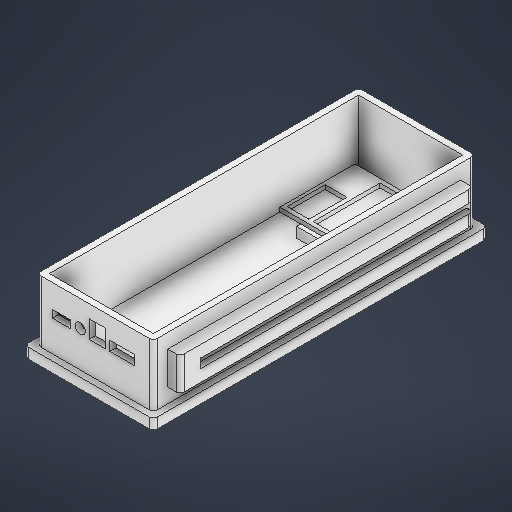
# Autodesk Inventor part: module_command
Saved by Autodesk Inventor 2025.2 (Build 292293000, 293)
## iProperties
Created: 2025-09-05
Part Number: module_command
Material: PC/ABS Plastic
Document SubType Name: Modeling
Designer: sam
Density: 1.1 g/cm^3
Appearance: Smooth - White
Author: sam
Autodesk Inventor part; units mm, degrees
ref_plane "YZ Plane" through (0, 0, 0) normal (1, 0, 0) x (0, 1, 0)
ref_plane "XZ Plane" through (0, 0, 0) normal (0, 1, 0) x (-1, 0, 0)
ref_plane "XY Plane" through (0, 0, 0) normal (0, 0, 1) x (1, 0, 0)
sketch "Sketch1" plane through (0, 0, 0) normal (0, 1, 0) x (-1, 0, 0)
  line L0 (-31.2, -81) -> (31.2, -81)
  line L1 (31.2, -81) -> (31.2, 81)
  line L2 (31.2, 81) -> (-31.2, 81)
  line L3 (-31.2, 81) -> (-31.2, -81)
  line L4 (-31.2, -81) -> (31.2, 81) construction
  line L5 (31.2, -81) -> (-31.2, 81) construction
  point P0 (0, 0)
  dimension "d0" = 62.4
  dimension "d1" = 162
  constraints: 12 end point, 2 midpoint, 2 parallel, 1 horizontal, 1 perpendicular
  measures "d0" distance of L2.end L1.end
  measures "d1" distance of L1.end L0.end
extrude "Extrusion1" add sketch "Sketch1" along normal blind 5
sketch "Sketch2" plane through (0, 5, 0) normal (0, 1, 0) x (1, 0, 0)
  line L0 (-31.2, 81) -> (-31.2, -81) projected
  line L1 (-31.2, -81) -> (31.2, -81) projected
  line L2 (31.2, -81) -> (31.2, 81) projected
  line L3 (31.2, 81) -> (-31.2, 81) projected
  line L4 (28.2, 78) -> (-28.2, 78)
  line L5 (-28.2, 78) -> (-28.2, -78)
  line L6 (-28.2, -78) -> (28.2, -78)
  line L7 (28.2, -78) -> (28.2, 78)
  line L8 (28.2, 78) -> (-28.2, -78) construction
  line L9 (-28.2, 78) -> (28.2, -78) construction
  line L10 (25.2, 75) -> (-25.2, 75)
  line L11 (-25.2, 75) -> (-25.2, -75)
  line L12 (-25.2, -75) -> (25.2, -75)
  line L13 (25.2, -75) -> (25.2, 75)
  line L14 (25.2, 75) -> (-25.2, -75) construction
  line L15 (-25.2, 75) -> (25.2, -75) construction
  point P0 (0, 0)
  dimension "d4" = 3
  dimension "d5" = 3
  dimension "d6" = 3
  dimension "d7" = 3
  constraints: 24 end point, 4 midpoint, 4 parallel, 2 horizontal, 2 perpendicular
  measures "d4" distance between parallel lines of L0 L5
  measures "d5" distance between parallel lines of L1 L6
  measures "d6" distance between parallel lines of L5 L11
  measures "d7" distance between parallel lines of L6 L12
extrude "Extrusion2" add sketch "Sketch2" along normal blind 30 contours L7 L6 L5 L4
fillet "Fillet1" radius 2 4 edges at (-28.2, 20, 78) (28.2, 20, 78) (28.2, 20, -78) (-28.2, 20, -78)
fillet "Fillet2" radius 2 4 edges at (-31.2, 2.5, 81) (31.2, 2.5, 81) (31.2, 2.5, -81) (-31.2, 2.5, -81)
sketch "Sketch3" plane through (28.2, 5, 76) normal (1, 0, 0) x (0, 0, -1)
  line L0 (152, 30) -> (152, 0) projected
  line L1 (0, 30) -> (152, 30) projected
  line L2 (0, 0) -> (0, 30) projected
  line L3 (152, 0) -> (0, 0) projected
  line L4 (5, 23) -> (147, 23)
  line L5 (147, 23) -> (147, 7)
  line L6 (147, 7) -> (5, 7)
  line L7 (5, 7) -> (5, 23)
  line L8 (-2, 30) -> (-2, 0) projected
  line L9 (154, 0) -> (154, 30) projected
  line L10 (157, -5) -> (157, 0) projected
  line L11 (-5, 0) -> (-5, -5) projected
  point P0 (76, -5)
  point P1 (147, 15)
  point P2 (-2, 15)
  dimension "d33" = 16
  dimension "d34" = 8
  dimension "d35" = 10
  dimension "d36" = 10
  constraints: 8 end point, 2 midpoint, 2 parallel, 1 horizontal, 1 perpendicular
  measures "d33" distance between parallel lines of L4 L6
  measures "d34" distance from line of L4 point (-2, 15)
  measures "d35" distance between parallel lines of L10 L5
  measures "d36" distance between parallel lines of L11 L7
extrude "Extrusion3" add sketch "Sketch3" along normal blind 6 contours L4 L5 L6 L7
sketch "Sketch4" plane through (28.2, 12, -71) normal (0, 0, -1) x (-1, 0, 0)
  line L0 (0, 16) -> (0, 0) projected
  line L1 (0, 16) -> (-6, 16) projected
  line L2 (-6, 0) -> (-6, 16) projected
  line L3 (0, 0) -> (-6, 0) projected
  line L4 (-6, 0) -> (-6, 16) projected
  line L5 (0, -7) -> (0, 23) projected
  line L6 (-6, 16) -> (0.4, 16)
  line L7 (0.4, 16) -> (0.4, 13.2)
  line L8 (0.4, 13.2) -> (-6, 13.2)
  line L9 (-6, 13.2) -> (-6, 16)
  line L10 (-6, 0) -> (0.4, 0)
  line L11 (0.4, 0) -> (0.4, 2.8)
  line L12 (0.4, 2.8) -> (-6, 2.8)
  line L13 (-6, 2.8) -> (-6, 0)
  line L14 (-6, 2.8) -> (-3, 2.8)
  line L15 (-3, 2.8) -> (-3, 5.8)
  line L16 (-3, 5.8) -> (-6, 5.8)
  line L17 (-6, 5.8) -> (-6, 2.8)
  line L18 (-6, 13.2) -> (-3, 13.2)
  line L19 (-3, 13.2) -> (-3, 10.2)
  line L20 (-3, 10.2) -> (-6, 10.2)
  line L21 (-6, 10.2) -> (-6, 13.2)
  point P0 (28.2, -12)
  point P1 (-6, 10.2)
  point P2 (-6, 5.8)
  point P3 (-3, 2.8)
  point P4 (0, 2.8)
  point P5 (0, 13.2)
  point P6 (-3, 13.2)
  point P7 (-6, 13.2)
  point P8 (0, 16)
  dimension "d102" = 6.4
  dimension "d103" = 2.8
  dimension "d104" = 6.4
  dimension "d105" = 2.8
  dimension "d106" = 3
  dimension "d107" = 3
  dimension "d108" = 3
  dimension "d109" = 3
  constraints: 32 end point, 8 parallel, 4 horizontal, 4 perpendicular
  measures "d102" distance of L7.end L8.end
  measures "d103" distance of L6.end L7.end
  measures "d104" distance of L12.end L11.end
  measures "d105" distance of L11.end L10.end
  measures "d106" distance of L16.end L15.end
  measures "d107" distance of L15.end L14.end
  measures "d108" distance of L19.end L20.end
  measures "d109" distance of L18.end L19.end
extrude "Extrusion4" cut sketch "Sketch4" against normal blind 132 contours L0 L12 L15 L16 L2 L20 L19 L8
fillet "Fillet3" radius 2 3 edges at (34.2, 20, 71) (34.2, 14.9, -71) (34.2, 25.1, -71)
sketch "Sketch5" plane through (-28.2, 5, -76) normal (-1, 0, 0) x (0, 0, 1)
  line L0 (0, 30) -> (152, 30) projected
  line L1 (-2, 30) -> (-2, 0) projected
  line L2 (154, 0) -> (154, 30) projected
  line L3 (5, 20) -> (137, 20)
  line L4 (137, 20) -> (137, 10)
  line L5 (137, 10) -> (5, 10)
  line L6 (5, 10) -> (5, 20)
  line L7 (-5, 0) -> (-5, -5) projected
  line L8 (157, -5) -> (157, 0) projected
  point P0 (76, -5)
  point P1 (154, 15)
  dimension "d28" = 10
  dimension "d39" = 10
  dimension "d40" = 20
  dimension "d41" = 5
  constraints: 8 end point, 2 parallel, 1 horizontal, 1 midpoint, 1 perpendicular
  measures "d28" distance of L3.end L4.end
  measures "d39" distance between parallel lines of L7 L6
  measures "d40" distance between parallel lines of L8 L4
  measures "d41" distance from line of point (154, 15) L3
extrude "Extrusion5" add sketch "Sketch5" along normal blind 6
sketch "Sketch6" plane through (-28.2, 15, 61) normal (0, 0, 1) x (1, 0, 0)
  line L0 (0, 10) -> (0, 0) projected
  line L1 (0, 10) -> (-6, 10) projected
  line L2 (-6, 0) -> (-6, 10) projected
  line L3 (0, 0) -> (-6, 0) projected
  line L4 (0, 10) -> (-3.4, 10)
  line L5 (-3.4, 10) -> (-3.4, 7)
  line L6 (-3.4, 7) -> (0, 7)
  line L7 (0, 7) -> (0, 10)
  line L8 (0, 0) -> (-3.4, 0)
  line L9 (-3.4, 0) -> (-3.4, 3)
  line L10 (-3.4, 3) -> (0, 3)
  line L11 (0, 3) -> (0, 0)
  point P0 (28.2, -15)
  point P1 (0, 3)
  point P2 (-3.4, 0)
  point P3 (0, 7)
  point P4 (-3.4, 10)
  dimension "d44" = 3.4
  dimension "d45" = 3
  dimension "d46" = 3.4
  dimension "d47" = 3
  constraints: 16 end point, 4 parallel, 2 horizontal, 2 perpendicular
  measures "d44" distance of L6.end L5.end
  measures "d45" distance of L5.end L4.end
  measures "d46" distance of L9.end L10.end
  measures "d47" distance of L8.end L9.end
extrude "Extrusion6" cut sketch "Sketch6" against normal up to surface (132 mm away) contours L0 L6 L5 L1 | L0 L3 L9 L10
fillet "Fillet4" radius 1 18 edges at (-34.2, 25, -5) (-31.6, 25, -5) (-34.2, 15, -5) (-31.6, 15, -5) (-34.2, 20, 61) (-31.6, 23.5, 61) (-32.9, 25, 61) (-32.9, 15, 61) (-31.6, 16.5, 61) (-31.6, 16.5, -71) (-34.2, 20, -71) (-31.6, 23.5, -71) (-32.9, 25, -71) (-32.9, 15, -71) (-29.9, 22, -71) (-29.9, 18, -71) (-29.9, 18, 61) (-29.9, 22, 61)
sketch "Sketch9" plane through (0, 5, 0) normal (0, 1, 0) x (1, 0, 0)
  line L0 (25.2, 75) -> (-25.2, 75) projected
  line L1 (-25.2, 75) -> (-25.2, -75) projected
  line L2 (-25.2, -75) -> (25.2, -75) projected
  line L3 (25.2, -75) -> (25.2, 75) projected
  line L4 (-25.2, -72.6) -> (25.2, -72.6)
  line L5 (25.2, -72.6) -> (25.2, -70.6)
  line L6 (25.2, -70.6) -> (-25.2, -70.6)
  line L7 (-25.2, -70.6) -> (-25.2, -72.6)
  line L8 (-25.2, 75) -> (-25.2, -75) projected
  line L9 (-25.2, 29.8) -> (25.2, 29.8)
  line L10 (25.2, 29.8) -> (25.2, 31.8)
  line L11 (25.2, 31.8) -> (-25.2, 31.8)
  line L12 (-25.2, 31.8) -> (-25.2, 29.8)
  line L13 (-25.2, 31.8) -> (-10.2, 31.8)
  line L14 (-10.2, 31.8) -> (-10.2, 29.8)
  line L15 (-10.2, 29.8) -> (-25.2, 29.8)
  line L16 (-25.2, 29.8) -> (-25.2, 31.8)
  point P0 (0, 0)
  point P1 (25.2, 17.2)
  point P2 (-25.2, 31.8)
  point P3 (25.2, 29.8)
  point P4 (-25.2, -70.6)
  point P5 (-10.2, 31.8)
  dimension "d79" = 2
  dimension "d80" = 2.4
  dimension "d81" = 2
  dimension "d82" = 100.4
  dimension "d87" = 15
  constraints: 24 end point, 6 parallel, 6 point on line, 3 horizontal, 3 perpendicular
  measures "d79" distance of L5.end L4.end
  measures "d80" distance between parallel lines of L2 L4
  measures "d81" distance of L10.end L9.end
  measures "d82" distance between parallel lines of L6 L9
  measures "d87" distance of L14.end L15.end
extrude "Extrusion9" add sketch "Sketch9" along normal blind 5 contours L3 L9 L14 L11 | L3 L4 L1 L6
sketch "Sketch10" plane through (0, 5, 0) normal (0, 1, 0) x (1, 0, 0)
  line L0 (-25.2, -70.6) -> (25.2, -70.6) projected
  line L1 (25.2, -70.6) -> (25.2, 29.8) projected
  line L2 (25.2, 29.8) -> (-10.2, 29.8) projected
  line L3 (-10.2, 29.8) -> (-10.2, 31.8) projected
  line L4 (-10.2, 31.8) -> (25.2, 31.8) projected
  line L5 (25.2, 31.8) -> (25.2, 75) projected
  line L6 (25.2, 75) -> (-25.2, 75) projected
  line L7 (-25.2, 75) -> (-25.2, -70.6) projected
  line L8 (-25.2, 36.8) -> (25.2, 36.8)
  line L9 (-25.2, 71.8) -> (-25.2, 36.8)
  line L10 (-25.2, 36.8) -> (25.2, 36.8)
  line L11 (25.2, 36.8) -> (25.2, 38.8)
  line L12 (25.2, 38.8) -> (-25.2, 38.8)
  line L13 (-25.2, 38.8) -> (-25.2, 36.8)
  line L14 (25.2, 31.8) -> (25.2, 75) projected
  line L15 (-25.2, 38.8) -> (25.2, 38.8)
  line L16 (25.2, 38.8) -> (25.2, 71.2)
  line L17 (25.2, 71.2) -> (-25.2, 71.2)
  line L18 (-25.2, 71.2) -> (25.2, 71.2)
  line L19 (25.2, 71.2) -> (25.2, 73.2)
  line L20 (25.2, 73.2) -> (-25.2, 73.2)
  line L21 (-25.2, 73.2) -> (-25.2, 71.2)
  line L22 (25.2, 38.8) -> (23.7, 38.8)
  line L23 (23.7, 38.8) -> (23.7, 71.2)
  line L24 (23.7, 71.2) -> (25.2, 71.2)
  line L25 (25.2, 71.2) -> (25.2, 38.8)
  line L26 (23.7, 38.8) -> (7.3, 38.8)
  line L27 (7.3, 38.8) -> (7.3, 71.2)
  line L28 (7.3, 71.2) -> (23.7, 71.2)
  line L29 (23.7, 71.2) -> (23.7, 38.8)
  line L30 (7.3, 38.8) -> (5.3, 38.8)
  line L31 (5.3, 38.8) -> (5.3, 71.2)
  line L32 (5.3, 71.2) -> (7.3, 71.2)
  line L33 (7.3, 71.2) -> (7.3, 38.8)
  line L34 (5.3, 38.8) -> (-11.1, 38.8)
  line L35 (-11.1, 38.8) -> (-11.1, 71.2)
  line L36 (-11.1, 71.2) -> (5.3, 71.2)
  line L37 (5.3, 71.2) -> (5.3, 38.8)
  line L38 (-11.1, 38.8) -> (-13.1, 38.8)
  line L39 (-13.1, 38.8) -> (-13.1, 71.2)
  line L40 (-13.1, 71.2) -> (-11.1, 71.2)
  line L41 (-11.1, 71.2) -> (-11.1, 38.8)
  line L42 (-25.2, 71.2) -> (-23.7, 71.2)
  line L43 (-23.7, 71.2) -> (-23.7, 38.8)
  line L44 (-23.7, 38.8) -> (-25.2, 38.8)
  line L45 (-25.2, 38.8) -> (-25.2, 71.2)
  line L46 (-23.7, 38.8) -> (-13.1, 38.8)
  line L47 (-13.1, 38.8) -> (-13.1, 57.2)
  line L48 (-13.1, 57.2) -> (-23.7, 57.2)
  line L49 (-23.7, 57.2) -> (-23.7, 38.8)
  point P0 (0, 0)
  point P1 (25.2, 36.8)
  point P2 (5.3, 38.8)
  point P3 (-11.1, 38.8)
  point P4 (-13.1, 38.8)
  point P5 (-23.7, 57.2)
  point P6 (23.7, 38.8)
  point P7 (7.3, 38.8)
  dimension "d89" = 5
  dimension "d90" = 2
  dimension "d91" = 32.4
  dimension "d92" = 2
  dimension "d93" = 1.5
  dimension "d94" = 16.4
  dimension "d95" = 2
  dimension "d96" = 16.4
  dimension "d97" = 2
  dimension "d98" = 1.5
  dimension "d99" = 18.4
  constraints: 82 end point, 19 parallel, 11 horizontal, 10 perpendicular, 10 point on line
  measures "d89" distance between parallel lines of L4 L8
  measures "d90" distance of L11.end L10.end
  measures "d91" distance of L16.end L15.end
  measures "d92" distance of L19.end L18.end
  measures "d93" distance of L23.end L24.end
  measures "d94" distance of L27.end L28.end
  measures "d95" distance of L31.end L32.end
  measures "d96" distance of L35.end L36.end
  measures "d97" distance of L39.end L40.end
  measures "d98" distance of L43.end L44.end
  measures "d99" distance of L47.end L46.end
extrude "Extrusion10" add sketch "Sketch10" along normal blind 2 contours L7 L12 L5 L8 | L7 L17 L43 L12 | L7 L20 L5 L17 | L12 L23 L17 L5 | L17 L39 L48 L43 | L39 L17 L35 L12 | L12 L31 L17 L27
sketch "Sketch11" plane through (-26.2, 5, 78) normal (0, 0, 1) x (1, 0, 0)
  line L0 (52.4, 30) -> (52.4, 0) projected
  line L1 (0, 30) -> (52.4, 30) projected
  line L2 (0, 0) -> (0, 30) projected
  line L3 (52.4, 0) -> (0, 0) projected
  line L4 (5.5, 15) -> (14.2, 15)
  line L5 (14.2, 15) -> (14.2, 18.7)
  line L6 (14.2, 18.7) -> (5.5, 18.7)
  line L7 (5.5, 18.7) -> (5.5, 15)
  line L8 (45.4, 15) -> (33.3, 15)
  line L9 (33.3, 15) -> (33.3, 19.7)
  line L10 (33.3, 19.7) -> (45.4, 19.7)
  line L11 (45.4, 19.7) -> (45.4, 15)
  circle A0 centre (19, 17.5) radius 2.5
  line L12 (-3, 0) -> (55.4, 0) projected
  line L13 (-2, 30) -> (-2, 0) projected
  line L14 (54.4, 0) -> (54.4, 30) projected
  line L15 (23.24, 15) -> (31.3, 15)
  line L16 (31.3, 15) -> (31.3, 23.7)
  line L17 (31.3, 23.7) -> (23.24, 23.7)
  line L18 (23.24, 23.7) -> (23.24, 15)
  point P0 (26.2, -5)
  dimension "d110" = 8.7
  dimension "d111" = 3.7
  dimension "d112" = 12.1
  dimension "d113" = 4.7
  dimension "d114" = 5
  dimension "d115" = 15
  dimension "d116" = 15
  dimension "d117" = 17.5
  dimension "d118" = 7.5
  dimension "d119" = 9
  dimension "d121" = 21
  dimension "d124" = 8.06
  dimension "d125" = 8.7
  dimension "d126" = 15
  dimension "d127" = 2
  constraints: 24 end point, 6 parallel, 3 horizontal, 3 perpendicular, 1 centre point
  measures "d110" distance of L6.end L5.end
  measures "d111" distance of L5.end L4.end
  measures "d112" distance of L9.end L10.end
  measures "d113" distance of L8.end L9.end
  measures "d114" diameter of A0
  measures "d115" distance between parallel lines of L12 L8
  measures "d116" distance between parallel lines of L3 L4
  measures "d117" distance from line of L3 A0.centre
  measures "d118" distance between parallel lines of L13 L7
  measures "d119" distance between parallel lines of L14 L11
  measures "d121" distance from line of L13 A0.centre
  measures "d124" distance of L17.end L16.end
  measures "d125" distance of L16.end L15.end
  measures "d126" distance between parallel lines of L3 L15
  measures "d127" distance between parallel lines of L16 L9
extrude "Extrusion11" cut sketch "Sketch11" against normal blind 3 contours L7 L6 L5 L4 | L8 L9 L10 L11 | A0 | L18 L17 L16 L15
body "Solid1"
